# Autodesk Inventor part: MAGJACK_RJ45
Saved by Autodesk Inventor 2015 SP1 (Build 190203100, 203)
## iProperties
Created: 2015-06-25
Part Number: MAGJACK_RJ45
Material: Generic
Document SubType Name: Modeling
Designer: Patrick
Density: 1 g/cm^3
Appearance: MAGJACKRJ45, MAGJACK_RJ45
Author: Patrick
Autodesk Inventor part; units mm, degrees
ref_plane "YZ Plane" through (0, 0, 0) normal (1, 0, 0) x (0, 1, 0)
ref_plane "XZ Plane" through (0, 0, 0) normal (0, 1, 0) x (-1, 0, 0)
ref_plane "XY Plane" through (0, 0, 0) normal (0, 0, 1) x (1, 0, 0)
sketch "MAGJACKRJ45, MAGJACK_RJ45_68" plane through (0, 0, 0) normal (0, 0, 1) x (1, 0, 0)
  line L0 (-8.747, -10.922) -> (-8.747, 10.922)
  line L1 (-8.747, 10.922) -> (8.747, 10.922)
  line L2 (8.747, 10.922) -> (8.747, -10.922)
  line L3 (8.747, -10.922) -> (-8.747, -10.922)
  constraints: 8 end point
extrude "Extrusion1" add sketch "MAGJACKRJ45, MAGJACK_RJ45_68" along normal blind 1
body "Solid1"
